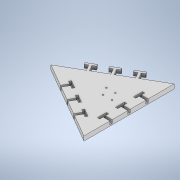
# Autodesk Inventor part: Base2
Saved by Autodesk Inventor 2022.3 (Build 263350000, 350)
## iProperties
Created: 2023-03-28
Part Number: Base2
Material: Generic
Document SubType Name: Modeling
Designer: Manuel Hueso Béjar
Density: 1 g/cm^3
Appearance: Default
Author: Manuel Hueso Béjar
Autodesk Inventor part; units mm, degrees
ref_plane "YZ Plane" through (0, 0, 0) normal (1, 0, 0) x (0, 1, 0)
ref_plane "XZ Plane" through (0, 0, 0) normal (0, 1, 0) x (-1, 0, 0)
ref_plane "XY Plane" through (0, 0, 0) normal (0, 0, 1) x (1, 0, 0)
sketch "Sketch1" plane through (0, 0, 0) normal (0, 1, 0) x (-1, 0, 0)
  circle A0 centre (0, 0) radius 115.4701
  line L0 (115.4701, 0) -> (-57.735, -100)
  line L1 (-57.735, -100) -> (-57.735, 100)
  line L2 (-57.735, 100) -> (115.4701, 0)
  line L3 (-40.235, 2.5) -> (-75.235, 2.5)
  line L4 (-75.235, 2.5) -> (-75.235, -2.5)
  line L5 (-75.235, -2.5) -> (-40.235, -2.5)
  line L6 (-40.235, -2.5) -> (-40.235, 2.5)
  line L7 (-40.235, 2.5) -> (-75.235, -2.5) construction
  line L8 (-75.235, 2.5) -> (-40.235, -2.5) construction
  line L9 (-42.735, 10) -> (-37.735, 10)
  line L10 (-37.735, 10) -> (-37.735, -10)
  line L11 (-37.735, -10) -> (-42.735, -10)
  line L12 (-42.735, -10) -> (-42.735, 10)
  line L13 (-42.735, 10) -> (-37.735, -10) construction
  line L14 (-37.735, 10) -> (-42.735, -10) construction
  line L15 (-37.735, 50) -> (-37.735, 30)
  line L16 (-42.735, 50) -> (-37.735, 50)
  line L17 (-42.735, 30) -> (-42.735, 50)
  line L18 (-37.735, 30) -> (-42.735, 30)
  line L19 (-40.235, 42.5) -> (-75.235, 42.5)
  line L20 (-75.235, 37.5) -> (-40.235, 37.5)
  line L21 (-37.735, 90) -> (-37.735, 70)
  line L22 (-42.735, 90) -> (-37.735, 90)
  line L23 (-42.735, 70) -> (-42.735, 90)
  line L24 (-37.735, 70) -> (-42.735, 70)
  line L25 (-40.235, 82.5) -> (-75.235, 82.5)
  line L26 (-75.235, 77.5) -> (-40.235, 77.5)
  line L27 (-37.735, -30) -> (-37.735, -50)
  line L28 (-42.735, -30) -> (-37.735, -30)
  line L29 (-42.735, -50) -> (-42.735, -30)
  line L30 (-37.735, -50) -> (-42.735, -50)
  line L31 (-40.235, -37.5) -> (-75.235, -37.5)
  line L32 (-75.235, -42.5) -> (-40.235, -42.5)
  line L33 (-37.735, 10) -> (-37.735, -10)
  line L34 (-42.735, 10) -> (-37.735, 10)
  line L35 (-42.735, -10) -> (-42.735, 10)
  line L36 (-37.735, -10) -> (-42.735, -10)
  line L37 (-40.235, 2.5) -> (-75.235, 2.5)
  line L38 (-75.235, -2.5) -> (-40.235, -2.5)
  line L39 (-37.735, 50) -> (-37.735, 30)
  line L40 (-42.735, 50) -> (-37.735, 50)
  line L41 (-42.735, 30) -> (-42.735, 50)
  line L42 (-37.735, 30) -> (-42.735, 30)
  line L43 (-40.235, 42.5) -> (-75.235, 42.5)
  line L44 (-75.235, 37.5) -> (-40.235, 37.5)
  line L45 (-37.735, -70) -> (-37.735, -90)
  line L46 (-42.735, -70) -> (-37.735, -70)
  line L47 (-42.735, -90) -> (-42.735, -70)
  line L48 (-37.735, -90) -> (-42.735, -90)
  line L49 (-40.235, -77.5) -> (-75.235, -77.5)
  line L50 (-75.235, -82.5) -> (-40.235, -82.5)
  line L51 (-37.735, -30) -> (-37.735, -50)
  line L52 (-42.735, -30) -> (-37.735, -30)
  line L53 (-42.735, -50) -> (-42.735, -30)
  line L54 (-37.735, -50) -> (-42.735, -50)
  line L55 (-40.235, -37.5) -> (-75.235, -37.5)
  line L56 (-75.235, -42.5) -> (-40.235, -42.5)
  line L57 (-37.735, 10) -> (-37.735, -10)
  line L58 (-42.735, 10) -> (-37.735, 10)
  line L59 (-42.735, -10) -> (-42.735, 10)
  line L60 (-37.735, -10) -> (-42.735, -10)
  line L61 (-40.235, 2.5) -> (-75.235, 2.5)
  line L62 (-75.235, -2.5) -> (-40.235, -2.5)
  point P0 (-57.735, 0)
  point P1 (-40.235, 0)
  point P2 (-42.735, 42.5)
  point P3 (-57.735, 42.5)
  point P4 (-57.735, 37.5)
  point P5 (-42.735, 37.5)
  point P6 (-42.735, -37.5)
  point P7 (-57.735, -37.5)
  point P8 (-57.735, -42.5)
  point P9 (-42.735, -42.5)
  point P10 (-42.735, 82.5)
  point P11 (-57.735, 82.5)
  point P12 (-57.735, 77.5)
  point P13 (-42.735, 77.5)
  point P14 (-42.735, -77.5)
  point P15 (-57.735, -77.5)
  point P16 (-57.735, -82.5)
  point P17 (-42.735, -82.5)
  point P18 (-42.735, -2.5)
  point P19 (-42.735, 2.5)
  point P20 (-57.735, 2.5)
  point P21 (-57.735, -2.5)
  point P22 (-40.4145, -90)
  point P23 (-37.735, -88.453)
  point P24 (-37.735, 88.453)
  point P25 (-40.4145, 90)
  dimension "d1" = 200
  dimension "d2" = 35
  dimension "d3" = 5
  dimension "d4" = 5
  dimension "d5" = 20
  dimension "d8" = 40
  dimension "d11" = 40
  constraints: 126 end point, 6 midpoint, 4 parallel, 2 coincident, 2 horizontal, 2 perpendicular, 2 vertical, 1 horizontal alignment, 121 other
  measures "d1" distance of L0.end L1.end
  measures "d2" distance of L5.end L4.end
  measures "d3" distance of L4.end L3.end
  measures "d4" distance of L10.end L11.end
  measures "d5" distance of L9.end L10.end
  measures "d8" distance of L9.end L15.start
  measures "d11" distance of L9.end L27.start
extrude "Extrusion1" add sketch "Sketch1" along normal blind 10 contours L0 L45 L46 L47 L49 L1 L32 L29 L30 L27 L28 L31 L5 L12 L11 L10 L9 L3 L20 L17 L18 L15 L16 L19 L26 L23 L24 L21 L2 | L2 L22 L23 L25 L1 | L1 L50 L47 L48 L0 | L0 L48 L47 L46 L45 | L21 L24 L23 L22 L2 | L25 L23 L26 L1 | L1 L49 L47 L50 | L19 L17 L20 L1 | L1 L31 L29 L32 | L17 L16 L15 L18 | L29 L28 L27 L30 | L3 L12 L5 L1 | L12 L9 L10 L11 L5 L6 L3 | L3 L6 L5 L12
extrude "Extrusion2" cut sketch "Sketch1" along normal blind 10 contours L19 L17 L20 L1 | L1 L31 L29 L32 | L17 L16 L15 L18 | L29 L28 L27 L30 | L3 L12 L5 L1 | L12 L9 L10 L11 L5 L6 L3 | L3 L6 L5 L12
extrude "Extrusion3" add sketch "Sketch1" along normal blind 2.5 contours L0 L48 L47 L46 L45 | L21 L24 L23 L22 L2 | L25 L23 L26 L1 | L1 L49 L47 L50 | L19 L17 L20 L1 | L1 L31 L29 L32 | L17 L16 L15 L18 | L29 L28 L27 L30 | L3 L12 L5 L1 | L12 L9 L10 L11 L5 L6 L3 | L3 L6 L5 L12
sketch "Sketch2" plane through (0, 0, 0) normal (0, -1, 0) x (1, 0, 0)
  line L0 (57.735, 100) -> (57.735, -100) projected
  line L1 (-115.4701, 0) -> (57.735, 100) projected
  line L2 (57.735, -100) -> (-115.4701, 0) projected
  line L3 (35.735, 61.8949) -> (35.735, -61.8949)
  line L4 (35.735, -61.8949) -> (-71.4701, 0)
  line L5 (-71.4701, 0) -> (35.735, 61.8949)
  line L6 (32.735, 56.6987) -> (32.735, -56.6987)
  line L7 (32.735, -56.6987) -> (-65.4701, 0)
  line L8 (-65.4701, 0) -> (32.735, 56.6987)
  point P0 (0, 0)
  dimension "d20" = 22
  dimension "d21" = 3
  constraints: 12 end point, 4 other
  measures "d20" distance between parallel lines of L1 L5
  measures "d21" distance between parallel lines of L5 L8
extrude "Extrusion4" cut sketch "Sketch2" against normal blind 1.5 contours L3 L4 L5
sketch "Sketch3" plane through (0, 10, 0) normal (0, 1, 0) x (1, 0, 0)
  line L0 (57.735, 100) -> (-115.4701, 0) projected
  line L1 (-28.8675, 50) -> (-36.3675, 62.9904)
  line L2 (-28.8675, 50) -> (-13.8675, 50) construction
  line L3 (-34.2024, 64.2404) -> (-27.7073, 67.9904)
  line L4 (-27.7073, 67.9904) -> (-30.2073, 72.3205)
  line L5 (-30.2073, 72.3205) -> (-47.5278, 62.3205)
  line L6 (-47.5278, 62.3205) -> (-45.0278, 57.9904)
  line L7 (-45.0278, 57.9904) -> (-38.5326, 61.7404)
  line L8 (-28.8675, 50) -> (-31.0326, 48.75)
  line L9 (-31.0326, 48.75) -> (-38.5326, 61.7404)
  line L10 (-31.0326, 48.75) -> (-26.7024, 51.25)
  line L11 (-26.7024, 51.25) -> (-34.2024, 64.2404)
  line L12 (-28.8675, -50) -> (-36.3675, -37.0096) construction
  line L13 (-28.8675, -50) -> (-26.7024, -51.25)
  line L14 (-26.7024, -51.25) -> (-31.0326, -48.75)
  line L15 (-28.8675, -50) -> (-36.3675, -62.9904)
  line L16 (-26.7024, -51.25) -> (-34.2024, -64.2404)
  line L17 (-31.0326, -48.75) -> (-38.5326, -61.7404)
  line L18 (-38.5326, -61.7404) -> (-45.0278, -57.9904)
  line L19 (-27.7073, -67.9904) -> (-34.2024, -64.2404)
  line L20 (-45.0278, -57.9904) -> (-47.5278, -62.3205)
  line L21 (-30.2073, -72.3205) -> (-27.7073, -67.9904)
  line L22 (-47.5278, -62.3205) -> (-30.2073, -72.3205)
  line L23 (-82.1688, 42.3205) -> (-79.6688, 37.9904)
  line L24 (-79.6688, 37.9904) -> (-73.1736, 41.7404)
  line L25 (-63.5085, 30) -> (-65.6736, 28.75)
  line L26 (-65.6736, 28.75) -> (-61.3435, 31.25)
  line L27 (-65.6736, 28.75) -> (-73.1736, 41.7404)
  line L28 (-63.5085, 30) -> (-71.0085, 42.9904)
  line L29 (-61.3435, 31.25) -> (-68.8435, 44.2404)
  line L30 (-64.8483, 52.3205) -> (-82.1688, 42.3205)
  line L31 (-63.5085, 30) -> (-48.5085, 30) construction
  line L32 (-62.3483, 47.9904) -> (-64.8483, 52.3205)
  line L33 (-68.8435, 44.2404) -> (-62.3483, 47.9904)
  line L34 (-116.8098, 22.3205) -> (-114.3098, 17.9904)
  line L35 (-114.3098, 17.9904) -> (-107.8146, 21.7404)
  line L36 (-98.1495, 10) -> (-100.3146, 8.75)
  line L37 (-100.3146, 8.75) -> (-95.9845, 11.25)
  line L38 (-100.3146, 8.75) -> (-107.8146, 21.7404)
  line L39 (-98.1495, 10) -> (-105.6495, 22.9904)
  line L40 (-95.9845, 11.25) -> (-103.4845, 24.2404)
  line L41 (-99.4893, 32.3205) -> (-116.8098, 22.3205)
  line L42 (-98.1495, 10) -> (-83.1495, 10) construction
  line L43 (-96.9893, 27.9904) -> (-99.4893, 32.3205)
  line L44 (-103.4845, 24.2404) -> (-96.9893, 27.9904)
  line L45 (-12.8868, 82.3205) -> (-10.3868, 77.9904)
  line L46 (-10.3868, 77.9904) -> (-3.8916, 81.7404)
  line L47 (5.7735, 70) -> (3.6084, 68.75)
  line L48 (3.6084, 68.75) -> (7.9386, 71.25)
  line L49 (3.6084, 68.75) -> (-3.8916, 81.7404)
  line L50 (5.7735, 70) -> (-1.7265, 82.9904)
  line L51 (7.9386, 71.25) -> (0.4386, 84.2404)
  line L52 (4.4338, 92.3205) -> (-12.8868, 82.3205)
  line L53 (5.7735, 70) -> (20.7735, 70) construction
  line L54 (6.9338, 87.9904) -> (4.4338, 92.3205)
  line L55 (0.4386, 84.2404) -> (6.9338, 87.9904)
  line L56 (-47.5278, 62.3205) -> (-45.0278, 57.9904)
  line L57 (-45.0278, 57.9904) -> (-38.5326, 61.7404)
  line L58 (-28.8675, 50) -> (-31.0326, 48.75)
  line L59 (-31.0326, 48.75) -> (-26.7024, 51.25)
  line L60 (-31.0326, 48.75) -> (-38.5326, 61.7404)
  line L61 (-28.8675, 50) -> (-36.3675, 62.9904)
  line L62 (-26.7024, 51.25) -> (-34.2024, 64.2404)
  line L63 (-30.2073, 72.3205) -> (-47.5278, 62.3205)
  line L64 (-28.8675, 50) -> (-13.8675, 50) construction
  line L65 (-27.7073, 67.9904) -> (-30.2073, 72.3205)
  line L66 (-34.2024, 64.2404) -> (-27.7073, 67.9904)
  line L67 (-82.1688, 42.3205) -> (-79.6688, 37.9904)
  line L68 (-79.6688, 37.9904) -> (-73.1736, 41.7404)
  line L69 (-63.5085, 30) -> (-65.6736, 28.75)
  line L70 (-65.6736, 28.75) -> (-61.3435, 31.25)
  line L71 (-65.6736, 28.75) -> (-73.1736, 41.7404)
  line L72 (-63.5085, 30) -> (-71.0085, 42.9904)
  line L73 (-61.3435, 31.25) -> (-68.8435, 44.2404)
  line L74 (-64.8483, 52.3205) -> (-82.1688, 42.3205)
  line L75 (-63.5085, 30) -> (-48.5085, 30) construction
  line L76 (-62.3483, 47.9904) -> (-64.8483, 52.3205)
  line L77 (-68.8435, 44.2404) -> (-62.3483, 47.9904)
  line L78 (21.7543, 102.3205) -> (24.2543, 97.9904)
  line L79 (24.2543, 97.9904) -> (30.7495, 101.7404)
  line L80 (40.4145, 90) -> (38.2495, 88.75)
  line L81 (38.2495, 88.75) -> (42.5796, 91.25)
  line L82 (38.2495, 88.75) -> (30.7495, 101.7404)
  line L83 (40.4145, 90) -> (32.9145, 102.9904)
  line L84 (42.5796, 91.25) -> (35.0796, 104.2404)
  line L85 (39.0748, 112.3205) -> (21.7543, 102.3205)
  line L86 (40.4145, 90) -> (55.4145, 90) construction
  line L87 (41.5748, 107.9904) -> (39.0748, 112.3205)
  line L88 (35.0796, 104.2404) -> (41.5748, 107.9904)
  line L89 (-12.8868, 82.3205) -> (-10.3868, 77.9904)
  line L90 (-10.3868, 77.9904) -> (-3.8916, 81.7404)
  line L91 (5.7735, 70) -> (3.6084, 68.75)
  line L92 (3.6084, 68.75) -> (7.9386, 71.25)
  line L93 (3.6084, 68.75) -> (-3.8916, 81.7404)
  line L94 (5.7735, 70) -> (-1.7265, 82.9904)
  line L95 (7.9386, 71.25) -> (0.4386, 84.2404)
  line L96 (4.4338, 92.3205) -> (-12.8868, 82.3205)
  line L97 (5.7735, 70) -> (20.7735, 70) construction
  line L98 (6.9338, 87.9904) -> (4.4338, 92.3205)
  line L99 (0.4386, 84.2404) -> (6.9338, 87.9904)
  line L100 (-47.5278, 62.3205) -> (-45.0278, 57.9904)
  line L101 (-45.0278, 57.9904) -> (-38.5326, 61.7404)
  line L102 (-28.8675, 50) -> (-31.0326, 48.75)
  line L103 (-31.0326, 48.75) -> (-26.7024, 51.25)
  line L104 (-31.0326, 48.75) -> (-38.5326, 61.7404)
  line L105 (-28.8675, 50) -> (-36.3675, 62.9904)
  line L106 (-26.7024, 51.25) -> (-34.2024, 64.2404)
  line L107 (-30.2073, 72.3205) -> (-47.5278, 62.3205)
  line L108 (-28.8675, 50) -> (-13.8675, 50) construction
  line L109 (-27.7073, 67.9904) -> (-30.2073, 72.3205)
  line L110 (-34.2024, 64.2404) -> (-27.7073, 67.9904)
  line L111 (-115.4701, 0) -> (57.735, -100) projected
  line L112 (57.735, -100) -> (-115.4701, 0)
  line L113 (5.7735, -70) -> (-1.7265, -57.0096) construction
  line L114 (5.7735, -70) -> (7.9386, -71.25)
  line L115 (7.9386, -71.25) -> (3.6084, -68.75)
  line L116 (3.6084, -68.75) -> (-3.8916, -81.7404)
  line L117 (5.7735, -70) -> (-1.7265, -82.9904)
  line L118 (7.9386, -71.25) -> (0.4386, -84.2404)
  line L119 (-3.8916, -81.7404) -> (-10.3868, -77.9904)
  line L120 (-10.3868, -77.9904) -> (-12.8868, -82.3205)
  line L121 (6.9338, -87.9904) -> (0.4386, -84.2404)
  line L122 (4.4338, -92.3205) -> (6.9338, -87.9904)
  line L123 (-12.8868, -82.3205) -> (4.4338, -92.3205)
  line L124 (40.4145, -90) -> (32.9145, -77.0096) construction
  line L125 (40.4145, -90) -> (42.5796, -91.25)
  line L126 (42.5796, -91.25) -> (38.2495, -88.75)
  line L127 (38.2495, -88.75) -> (30.7495, -101.7404)
  line L128 (40.4145, -90) -> (32.9145, -102.9904)
  line L129 (42.5796, -91.25) -> (35.0796, -104.2404)
  line L130 (30.7495, -101.7404) -> (24.2543, -97.9904)
  line L131 (24.2543, -97.9904) -> (21.7543, -102.3205)
  line L132 (41.5748, -107.9904) -> (35.0796, -104.2404)
  line L133 (39.0748, -112.3205) -> (41.5748, -107.9904)
  line L134 (21.7543, -102.3205) -> (39.0748, -112.3205)
  line L135 (-63.5085, -30) -> (-71.0085, -17.0096) construction
  line L136 (-63.5085, -30) -> (-61.3435, -31.25)
  line L137 (-61.3435, -31.25) -> (-65.6736, -28.75)
  line L138 (-65.6736, -28.75) -> (-73.1736, -41.7404)
  line L139 (-63.5085, -30) -> (-71.0085, -42.9904)
  line L140 (-61.3435, -31.25) -> (-68.8435, -44.2404)
  line L141 (-73.1736, -41.7404) -> (-79.6688, -37.9904)
  line L142 (-79.6688, -37.9904) -> (-82.1688, -42.3205)
  line L143 (-62.3483, -47.9904) -> (-68.8435, -44.2404)
  line L144 (-64.8483, -52.3205) -> (-62.3483, -47.9904)
  line L145 (-82.1688, -42.3205) -> (-64.8483, -52.3205)
  line L146 (-28.8675, -50) -> (-36.3675, -37.0096) construction
  line L147 (-28.8675, -50) -> (-26.7024, -51.25)
  line L148 (-26.7024, -51.25) -> (-31.0326, -48.75)
  line L149 (-31.0326, -48.75) -> (-38.5326, -61.7404)
  line L150 (-28.8675, -50) -> (-36.3675, -62.9904)
  line L151 (-26.7024, -51.25) -> (-34.2024, -64.2404)
  line L152 (-38.5326, -61.7404) -> (-45.0278, -57.9904)
  line L153 (-45.0278, -57.9904) -> (-47.5278, -62.3205)
  line L154 (-27.7073, -67.9904) -> (-34.2024, -64.2404)
  line L155 (-30.2073, -72.3205) -> (-27.7073, -67.9904)
  line L156 (-47.5278, -62.3205) -> (-30.2073, -72.3205)
  line L157 (5.7735, -70) -> (-1.7265, -57.0096) construction
  line L158 (5.7735, -70) -> (7.9386, -71.25)
  line L159 (7.9386, -71.25) -> (3.6084, -68.75)
  line L160 (3.6084, -68.75) -> (-3.8916, -81.7404)
  line L161 (5.7735, -70) -> (-1.7265, -82.9904)
  line L162 (7.9386, -71.25) -> (0.4386, -84.2404)
  line L163 (-3.8916, -81.7404) -> (-10.3868, -77.9904)
  line L164 (-10.3868, -77.9904) -> (-12.8868, -82.3205)
  line L165 (6.9338, -87.9904) -> (0.4386, -84.2404)
  line L166 (4.4338, -92.3205) -> (6.9338, -87.9904)
  line L167 (-12.8868, -82.3205) -> (4.4338, -92.3205)
  line L168 (-98.1495, -10) -> (-105.6495, 2.9904) construction
  line L169 (-98.1495, -10) -> (-95.9845, -11.25)
  line L170 (-95.9845, -11.25) -> (-100.3146, -8.75)
  line L171 (-100.3146, -8.75) -> (-107.8146, -21.7404)
  line L172 (-98.1495, -10) -> (-105.6495, -22.9904)
  line L173 (-95.9845, -11.25) -> (-103.4845, -24.2404)
  line L174 (-107.8146, -21.7404) -> (-114.3098, -17.9904)
  line L175 (-114.3098, -17.9904) -> (-116.8098, -22.3205)
  line L176 (-96.9893, -27.9904) -> (-103.4845, -24.2404)
  line L177 (-99.4893, -32.3205) -> (-96.9893, -27.9904)
  line L178 (-116.8098, -22.3205) -> (-99.4893, -32.3205)
  line L179 (-63.5085, -30) -> (-71.0085, -17.0096) construction
  line L180 (-63.5085, -30) -> (-61.3435, -31.25)
  line L181 (-61.3435, -31.25) -> (-65.6736, -28.75)
  line L182 (-65.6736, -28.75) -> (-73.1736, -41.7404)
  line L183 (-63.5085, -30) -> (-71.0085, -42.9904)
  line L184 (-61.3435, -31.25) -> (-68.8435, -44.2404)
  line L185 (-73.1736, -41.7404) -> (-79.6688, -37.9904)
  line L186 (-79.6688, -37.9904) -> (-82.1688, -42.3205)
  line L187 (-62.3483, -47.9904) -> (-68.8435, -44.2404)
  line L188 (-64.8483, -52.3205) -> (-62.3483, -47.9904)
  line L189 (-82.1688, -42.3205) -> (-64.8483, -52.3205)
  line L190 (-28.8675, -50) -> (-36.3675, -37.0096) construction
  line L191 (-28.8675, -50) -> (-26.7024, -51.25)
  line L192 (-26.7024, -51.25) -> (-31.0326, -48.75)
  line L193 (-31.0326, -48.75) -> (-38.5326, -61.7404)
  line L194 (-28.8675, -50) -> (-36.3675, -62.9904)
  line L195 (-26.7024, -51.25) -> (-34.2024, -64.2404)
  line L196 (-38.5326, -61.7404) -> (-45.0278, -57.9904)
  line L197 (-45.0278, -57.9904) -> (-47.5278, -62.3205)
  line L198 (-27.7073, -67.9904) -> (-34.2024, -64.2404)
  line L199 (-30.2073, -72.3205) -> (-27.7073, -67.9904)
  line L200 (-47.5278, -62.3205) -> (-30.2073, -72.3205)
  line L201 (-28.8675, -50) -> (-43.8675, -50) construction
  line L202 (-28.8675, -50) -> (-21.3675, -37.0096)
  line L203 (-26.7024, -51.25) -> (-19.2024, -38.2596)
  line L204 (-31.0326, -48.75) -> (-23.5326, -35.7596)
  line L205 (-23.5326, -35.7596) -> (-30.0278, -32.0096)
  line L206 (-12.7073, -42.0096) -> (-19.2024, -38.2596)
  line L207 (-30.0278, -32.0096) -> (-27.5278, -27.6795)
  line L208 (-10.2073, -37.6795) -> (-12.7073, -42.0096)
  line L209 (-27.5278, -27.6795) -> (-10.2073, -37.6795)
  line L210 (5.7735, -70) -> (-9.2265, -70) construction
  line L211 (3.6084, -68.75) -> (11.1084, -55.7596)
  line L212 (5.7735, -70) -> (13.2735, -57.0096)
  line L213 (7.9386, -71.25) -> (15.4386, -58.2596)
  line L214 (11.1084, -55.7596) -> (4.6132, -52.0096)
  line L215 (4.6132, -52.0096) -> (7.1132, -47.6795)
  line L216 (21.9338, -62.0096) -> (15.4386, -58.2596)
  line L217 (24.4338, -57.6795) -> (21.9338, -62.0096)
  line L218 (7.1132, -47.6795) -> (24.4338, -57.6795)
  line L219 (40.4145, -90) -> (25.4145, -90) construction
  line L220 (38.2495, -88.75) -> (45.7495, -75.7596)
  line L221 (40.4145, -90) -> (47.9145, -77.0096)
  line L222 (42.5796, -91.25) -> (50.0796, -78.2596)
  line L223 (45.7495, -75.7596) -> (39.2543, -72.0096)
  line L224 (39.2543, -72.0096) -> (41.7543, -67.6795)
  line L225 (56.5748, -82.0096) -> (50.0796, -78.2596)
  line L226 (59.0748, -77.6795) -> (56.5748, -82.0096)
  line L227 (41.7543, -67.6795) -> (59.0748, -77.6795)
  line L228 (-63.5085, -30) -> (-78.5085, -30) construction
  line L229 (-65.6736, -28.75) -> (-58.1736, -15.7596)
  line L230 (-63.5085, -30) -> (-56.0085, -17.0096)
  line L231 (-61.3435, -31.25) -> (-53.8435, -18.2596)
  line L232 (-58.1736, -15.7596) -> (-64.6688, -12.0096)
  line L233 (-64.6688, -12.0096) -> (-62.1688, -7.6795)
  line L234 (-47.3483, -22.0096) -> (-53.8435, -18.2596)
  line L235 (-44.8483, -17.6795) -> (-47.3483, -22.0096)
  line L236 (-62.1688, -7.6795) -> (-44.8483, -17.6795)
  line L237 (-28.8675, -50) -> (-43.8675, -50) construction
  line L238 (-31.0326, -48.75) -> (-23.5326, -35.7596)
  line L239 (-28.8675, -50) -> (-21.3675, -37.0096)
  line L240 (-26.7024, -51.25) -> (-19.2024, -38.2596)
  line L241 (-23.5326, -35.7596) -> (-30.0278, -32.0096)
  line L242 (-30.0278, -32.0096) -> (-27.5278, -27.6795)
  line L243 (-12.7073, -42.0096) -> (-19.2024, -38.2596)
  line L244 (-10.2073, -37.6795) -> (-12.7073, -42.0096)
  line L245 (-27.5278, -27.6795) -> (-10.2073, -37.6795)
  line L246 (5.7735, -70) -> (-9.2265, -70) construction
  line L247 (3.6084, -68.75) -> (11.1084, -55.7596)
  line L248 (5.7735, -70) -> (13.2735, -57.0096)
  line L249 (7.9386, -71.25) -> (15.4386, -58.2596)
  line L250 (11.1084, -55.7596) -> (4.6132, -52.0096)
  line L251 (4.6132, -52.0096) -> (7.1132, -47.6795)
  line L252 (21.9338, -62.0096) -> (15.4386, -58.2596)
  line L253 (24.4338, -57.6795) -> (21.9338, -62.0096)
  line L254 (7.1132, -47.6795) -> (24.4338, -57.6795)
  line L255 (-98.1495, -10) -> (-113.1495, -10) construction
  line L256 (-100.3146, -8.75) -> (-92.8146, 4.2404)
  line L257 (-98.1495, -10) -> (-90.6495, 2.9904)
  line L258 (-95.9845, -11.25) -> (-88.4845, 1.7404)
  line L259 (-92.8146, 4.2404) -> (-99.3098, 7.9904)
  line L260 (-99.3098, 7.9904) -> (-96.8098, 12.3205)
  line L261 (-81.9893, -2.0096) -> (-88.4845, 1.7404)
  line L262 (-79.4893, 2.3205) -> (-81.9893, -2.0096)
  line L263 (-96.8098, 12.3205) -> (-79.4893, 2.3205)
  line L264 (-63.5085, -30) -> (-78.5085, -30) construction
  line L265 (-65.6736, -28.75) -> (-58.1736, -15.7596)
  line L266 (-63.5085, -30) -> (-56.0085, -17.0096)
  line L267 (-61.3435, -31.25) -> (-53.8435, -18.2596)
  line L268 (-58.1736, -15.7596) -> (-64.6688, -12.0096)
  line L269 (-64.6688, -12.0096) -> (-62.1688, -7.6795)
  line L270 (-47.3483, -22.0096) -> (-53.8435, -18.2596)
  line L271 (-44.8483, -17.6795) -> (-47.3483, -22.0096)
  line L272 (-62.1688, -7.6795) -> (-44.8483, -17.6795)
  line L273 (-28.8675, -50) -> (-43.8675, -50) construction
  line L274 (-31.0326, -48.75) -> (-23.5326, -35.7596)
  line L275 (-28.8675, -50) -> (-21.3675, -37.0096)
  line L276 (-26.7024, -51.25) -> (-19.2024, -38.2596)
  line L277 (-23.5326, -35.7596) -> (-30.0278, -32.0096)
  line L278 (-30.0278, -32.0096) -> (-27.5278, -27.6795)
  line L279 (-12.7073, -42.0096) -> (-19.2024, -38.2596)
  line L280 (-10.2073, -37.6795) -> (-12.7073, -42.0096)
  line L281 (-27.5278, -27.6795) -> (-10.2073, -37.6795)
  point P0 (0, 0)
  point P1 (3.6084, 68.75)
  point P2 (7.9386, 71.25)
  point P3 (-65.6736, 28.75)
  point P4 (-61.3435, 31.25)
  point P5 (-100.3146, 8.75)
  point P6 (-95.9845, 11.25)
  point P7 (42.5796, -91.25)
  point P8 (38.2495, -88.75)
  point P9 (7.9386, -71.25)
  point P10 (3.6084, -68.75)
  point P11 (-61.3435, -31.25)
  point P12 (-65.6736, -28.75)
  point P13 (-95.9845, -11.25)
  point P14 (-100.3146, -8.75)
  point P15 (7.9386, -71.25)
  point P16 (3.6084, -68.75)
  point P17 (-12.7073, -42.0096)
  point P18 (-65.6736, -28.75)
  point P19 (-61.3435, -31.25)
  dimension "d24" = 15
  dimension "d25" = 120
  dimension "d26" = 10
  dimension "d27" = 5
  dimension "d28" = 20
  dimension "d29" = 90
  dimension "d30" = 5
  dimension "d31" = 2.5
  dimension "d32" = 5
  dimension "d35" = 120
  dimension "d39" = 40
  dimension "d42" = 40
  dimension "d47" = 40
  dimension "d50" = 40
  constraints: 560 end point, 72 symmetric about line, 6 perpendicular, 2 point on line, 1 collinear, 1 equal length, 1 horizontal, 1 midpoint, 379 other
  measures "d24" distance of L1.start L1.end
  measures "d25" angle of L2 L1
  measures "d26" distance of L1.end L3.end
  measures "d27" distance of L3.end L4.end
  measures "d28" distance of L4.end L5.end
  measures "d29" angle of L5 L4
  measures "d30" distance of L5.end L6.end
  measures "d31" distance of L1.start L8.end
  measures "d32" distance of L8.end L10.end
  measures "d39" distance of L6.end L23.end
  measures "d42" distance of L6.end L45.end
  measures "d47" distance of L12.end L113.end
  measures "d50" distance of L12.end L135.end
extrude "Extrusion6" cut sketch "Sketch3" against normal up to surface (7.5 mm away) contours L14 L204 L205 L207 L209 L208 L206 L203 L13 | L229 L232 L233 L236 L235 L234 L231 L111 | L211 L214 L215 L218 L217 L216 L213 L111
extrude "Extrusion7" add sketch "Sketch3" against normal up to surface (7.5 mm away) contours L0 L49 L46 L45 L52 L54 L55 L51 | L0 L9 L7 L6 L5 L4 L3 L11 | L0 L27 L24 L23 L30 L32 L33 L29
sketch "Sketch4" plane through (0, 10, 0) normal (0, 1, 0) x (1, 0, 0)
  line L0 (-115.4701, 0) -> (57.735, 0)
  line L1 (57.735, -100) -> (57.735, 100) projected
  line L2 (57.735, -100) -> (-28.8675, 50)
  line L3 (57.735, 100) -> (-115.4701, 0) projected
  line L4 (57.735, 100) -> (-28.8675, -50)
  line L5 (-115.4701, 0) -> (57.735, -100) projected
  circle A0 centre (0, 0) radius 20
  line L6 (10, 17.3205) -> (20, 0)
  line L7 (20, 0) -> (10, -17.3205)
  line L8 (10, -17.3205) -> (-10, -17.3205)
  line L9 (-10, -17.3205) -> (-20, 0)
  line L10 (-20, 0) -> (-10, 17.3205)
  line L11 (-10, 17.3205) -> (10, 17.3205)
  dimension "d59" = 40
  constraints: 18 end point, 3 midpoint, 2 coincident, 1 point on line, 16 other
hole "Hole1" at (0, 10, 0) at (-10, 10, -17.3205) at (20, 10, 0) at (10, 10, -17.3205) direction (0, -1, 0) diameter 2.2 depth 6.3 counterbore diameter 3.1 counterbore depth 4.1
body "Solid1"
